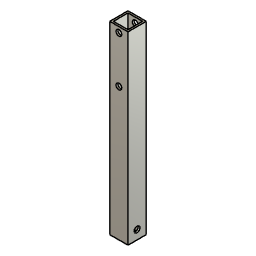
potention_pole (Autodesk Fusion 360 design; units mm, degrees)
Autodesk Fusion 360 part; units mm, degrees
sketch "スケッチ1" plane through (0, 0, 0) normal (0, 1, 0) x (1, 0, 0)
  line L0 (0, 0) -> (10, 0)
  line L1 (10, 0) -> (10, -10)
  line L2 (10, -10) -> (0, -10)
  line L3 (0, -10) -> (0, 0)
  line L4 (1, -1) -> (9, -1)
  line L5 (9, -1) -> (9, -9)
  line L6 (9, -9) -> (1, -9)
  line L7 (1, -9) -> (1, -1)
  dimension "d1" = 10
  dimension "d2" = 10
  dimension "d3" = 8
  dimension "d4" = 8
  constraint horizontal L0
  constraint vertical L1
  constraint horizontal L2
  constraint vertical L3
  constraint coincident L0.start L3.end
  constraint horizontal L4
  constraint vertical L5
  constraint horizontal L6
  constraint vertical L7
  measures "d1" distance of L0.start L0.end
  measures "d2" distance of L0.start L2.end
  measures "d3" distance of L4.start L4.end
  measures "d4" distance of L4.start L6.end
extrude "押し出し1" add sketch "スケッチ1" along normal blind 100 makes body 1
sketch "スケッチ2" plane through (0, 0, 10) normal (0, 0, 1) x (1, 0, 0)
  line L0 (0, 0) -> (10, 0)
  line L1 (10, 0) -> (10, 100)
  line L2 (10, 100) -> (0, 100)
  line L3 (0, 100) -> (0, 0)
  point P0 (5, 73)
  dimension "d7" = 73
  measures "d7" distance of L0 P0
hole "穴1" at (5, 73, 10) direction (0, 0, -1) diameter 3.2 depth 100 tip angle 118 bodies 1
sketch "スケッチ3" plane through (10, 0, 0) normal (1, 0, 0) x (0, 0, -1)
  line L0 (-10, 0) -> (0, 0)
  line L1 (0, 0) -> (0, 100)
  line L2 (0, 100) -> (-10, 100)
  line L3 (-10, 100) -> (-10, 0)
  point P0 (-5, 5)
  dimension "d11" = 5
  measures "d11" distance of L0 P0
hole "穴2" at (10, 5, 5) direction (-1, 0, 0) diameter 3.2 depth 100 tip angle 118 bodies 1
sketch "スケッチ4" plane through (0, 0, 10) normal (0, 0, 1) x (1, 0, 0)
  circle A0 centre (5, 73) radius 1.6
  line L0 (0, 0) -> (10, 0)
  line L1 (10, 0) -> (10, 100)
  line L2 (10, 100) -> (0, 100)
  line L3 (0, 100) -> (0, 0)
  point P0 (5, 97)
  dimension "d15" = 3
  measures "d15" distance of L2 P0
hole "穴3" at (5, 97, 10) direction (0, 0, -1) diameter 3.2 depth 100 tip angle 118 bodies 1
move_face "面を移動1" to x (1, 0, 0) y (0, 1, 0) z (0, 0, 1) at (0, 1, 0) 2 faces at (3.4005, 97.0399, 0.6667) (3.4005, 97.0399, 9.6667) on bodies 1
extrude "押し出し2" add 1 faces at (0.3333, 100, 3.6667) along direction (0, 1, 0) blind 1 on bodies 1 bodies 1
move_face "面を移動2" to x (1, 0, 0) y (0, 1, 0) z (0, 0, 1) at (0, 1, 0) 2 faces at (3.4005, 98.0399, 0.6667) (3.4005, 98.0399, 9.6667) on bodies 1
extrude "押し出し3" add 1 faces at (0.3333, 101, 3.6667) along direction (0, 1, 0) blind 1 on bodies 1 bodies 1
move_face "面を移動3" to x (1, 0, 0) y (0, 1, 0) z (0, 0, 1) at (0, -0.5, 0) 2 faces at (3.4005, 99.0399, 0.6667) (3.4005, 99.0399, 9.6667) on bodies 1
extrude "押し出し4" cut 1 faces at (0.3333, 102, 3.6667) along direction (0, -1, 0) blind 0.5 on bodies 1 bodies 1
copy_body "ボディ -> コンポーネント1" bodies 1 removing the originals makes body 2 in component "Component"
component "Component" placed x (1, 0, 0) y (0, 1, 0) z (0, 0, 1) at (0, 0, 0)
